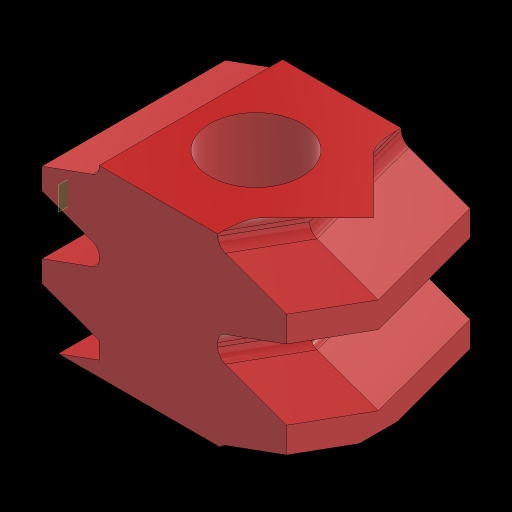
# Autodesk Inventor part: rack
Saved by Autodesk Inventor 2023.2 (Build 272271030, 271C)
## iProperties
Created: 2023-10-23
Part Number: rack
Material: Generic
Document SubType Name: Modeling
Designer: robpl
Density: 1 g/cm^3
Appearance: Red
Author: robpl
## iProperties of the stored document rack_3DPrint.ipt
Created: 2023-10-23
Part Number: rack_3DPrint
Material: Generic
Document SubType Name: Modeling
Designer: robpl
Density: 1 g/cm^3
Appearance: Default
Author: robpl
Autodesk Inventor part; units mm, degrees
ref_plane "YZ Plane" through (0, 0, 0) normal (1, 0, 0) x (0, 1, 0)
ref_plane "XZ Plane" through (0, 0, 0) normal (0, 1, 0) x (-1, 0, 0)
ref_plane "XY Plane" through (0, 0, 0) normal (0, 0, 1) x (1, 0, 0)
sketch "Sketch1" plane through (0, 0, 0) normal (0, 0, 1) x (1, 0, 0)
  line L0 (-6, -4.5) -> (6, -4.5)
  line L1 (6, -4.5) -> (6, 4.5)
  line L2 (6, 4.5) -> (-6, 4.5)
  line L3 (-6, 4.5) -> (-6, -4.5)
  point P0 (0, 0)
  point P1 (-6, 0)
  point P2 (0, 4.5)
  dimension "d0" = 12
  dimension "d1" = 9
  constraints: 8 end point, 2 midpoint, 2 parallel, 1 horizontal, 1 horizontal alignment, 1 perpendicular, 1 vertical alignment
  measures "d0" distance of L2.end L1.end
  measures "d1" distance of L1.end L0.end
extrude "Extrusion1" add sketch "Sketch1" along normal blind 4.5
sketch "Sketch2" plane through (0, 0, 4.5) normal (0, 0, 1) x (1, 0, 0)
  line L0 (6, -4.5) -> (6, 4.5) projected
  line L1 (6, 4.5) -> (-6, 4.5) projected
  line L2 (-6, 4.5) -> (-6, -4.5) projected
  line L3 (-6, -4.5) -> (6, -4.5) projected
  line L4 (6, -4.5) -> (6, 4.5) projected
  line L5 (6, 6.2241) -> (2.625, 4.9957)
  line L6 (2.625, 4.9957) -> (2.625, 4.0043)
  line L7 (2.625, 4.0043) -> (6, 2.7759)
  line L8 (6, 1.5117) -> (2.625, 0.2833)
  line L9 (2.625, 0.2833) -> (2.625, -0.708)
  line L10 (2.625, -0.708) -> (6, -1.9364)
  arc A0 (3, 5.1322) -> (2.625, 4.5965) centre (3.195, 4.5965) ccw
  arc A1 (2.625, 4.4035) -> (3, 3.8678) centre (3.195, 4.4035) ccw
  line L11 (6, 4.5) -> (-6, 4.5) projected
  arc A2 (2.625, -0.3089) -> (3, -0.8445) centre (3.195, -0.3089) ccw
  arc A3 (3, 0.4198) -> (2.625, -0.1159) centre (3.195, -0.1159) ccw
  line L12 (6, 6.2241) -> (6, 2.7759)
  line L13 (0, 4.5) -> (1.3125, -4.5)
  line L14 (0, -4.5) -> (6, -4.5) projected
  line L15 (-6.2425, 4.4387) -> (-2.6572, 4.2253)
  line L16 (-2.6572, 4.2253) -> (-2.3741, 3.2753)
  line L17 (-2.3741, 3.2753) -> (-5.2577, 1.1342)
  arc A4 (-2.5432, 3.8428) -> (-3.0556, 4.249) centre (-3.0895, 3.68) ccw
  arc A5 (-2.6946, 3.0374) -> (-2.4881, 3.6578) centre (-3.0344, 3.495) ccw
  line L18 (-6.2425, 4.4387) -> (-5.2577, 1.1342)
  line L19 (-4.8967, -0.0774) -> (-1.3114, -0.2908)
  line L20 (-1.3114, -0.2908) -> (-1.0283, -1.2408)
  line L21 (-1.0283, -1.2408) -> (-3.9119, -3.3819)
  arc A6 (-1.3487, -1.4787) -> (-1.1423, -0.8583) centre (-1.6885, -1.0211) ccw
  arc A7 (-1.1974, -0.6733) -> (-1.7098, -0.2671) centre (-1.7437, -0.8361) ccw
  point P0 (0, 0)
  point P1 (0, 0)
  point P2 (2.625, 4.5)
  point P3 (4.5, 3.3219)
  point P4 (4.5, 0.9657)
  point P5 (6, 2.7759)
  point P6 (2.625, 4.5)
  point P7 (6, -1.9364)
  point P8 (6, 1.5117)
  point P9 (6, 4.5)
  point P10 (-2.5157, 3.7503)
  point P11 (-3.9761, 2.0858)
  point P12 (-6, 3.625)
  point P13 (0, 7.2759)
  point P14 (-3.3032, -0.1723)
  point P15 (0, 2.5636)
  point P16 (0, 6.0117)
  point P17 (4.5, -1.3905)
  dimension "d14" = 70
  dimension "d15" = 4.7124
  dimension "d16" = 0.57
  dimension "d17" = 3.375
  dimension "d18" = 1.5
  dimension "d19" = 2.3562
  dimension "d48" = 2.3562
  constraints: 30 end point, 26 point on line, 23 symmetric about line, 16 point on circle, 8 centre point, 8 tangent, 4 equal length, 3 equal radius, 2 midpoint, 2 vertical, 2 vertical alignment, 1 parallel, 6 other
  measures "d14" angle of L0 L5
  measures "d15" distance of L10.end L7.end
  measures "d16" radius of A0
  measures "d17" distance between parallel lines of L6 L0
  measures "d18" distance from line of L0 point (4.5, 3.322)
  measures "d19" distance of point (4.5, 3.322) point (4.5, 0.966)
  measures "d48" distance of point (4.5, 0.966) point (4.5, -1.39)
sketch "Sketch3" plane through (6, -4.5, 0) normal (1, 0, 0) x (0, 0, -1)
  line L0 (-4.5, 0) -> (-4.5, 9) projected
  line L1 (-4.5, 9) -> (-4.5, 0) projected
  line L2 (-4.5, 2.5636) -> (0, 0.9257)
  line L3 (0, 4.5) -> (0, 9) projected
  line L4 (0, 9) -> (-4.5, 9) projected
  dimension "d31" = 20
  constraints: 2 end point, 1 point on line
  measures "d31" angle of L4 L2
sweep "Sweep1" cut profiles "Sketch2" path "Sketch3" path curves L2 contours L10 A2 L9 A3 L8 L0 | L7 A1 L6 L1 L0 | L6 A0 L5 L12 L1
pattern_linear "Rectangular Pattern2" count 8 spacing 4.7124 along (0, -1, 0) of "Sweep1"
mirror "Mirror2" about plane through (0, 0, 0) normal (0, 0, -1)
ref_plane "Work Plane3" through (4.5, 2.8745, 4.5) normal (1, 0, 0) x (0, 0, -1)
sketch "Sketch6" plane through (0, 0, 4.5) normal (0, 0, 1) x (1, 0, 0)
  arc A0 (3, -4.2926) -> (2.729, -4.5) centre (3.195, -4.8283) ccw projected
  line L0 (3, -4.2926) -> (6, -3.2007) projected
  line L1 (6, -3.2007) -> (6, -1.9364) projected
  line L2 (6, -1.9364) -> (3, -0.8445) projected
  arc A1 (2.625, -0.3089) -> (3, -0.8445) centre (3.195, -0.3089) ccw projected
  line L3 (2.625, -0.3089) -> (2.625, -0.1159) projected
  arc A2 (3, 0.4198) -> (2.625, -0.1159) centre (3.195, -0.1159) ccw projected
  line L4 (3, 0.4198) -> (6, 1.5117) projected
  line L5 (6, 1.5117) -> (6, 2.7759) projected
  line L6 (6, 2.7759) -> (3, 3.8678) projected
  arc A3 (2.625, 4.4035) -> (3, 3.8678) centre (3.195, 4.4035) ccw projected
  line L7 (2.625, 4.4035) -> (2.625, 4.5) projected
  line L8 (2.625, 4.5) -> (-6, 4.5) projected
  line L9 (-6, 4.5) -> (-6, -4.5) projected
  line L10 (-6, -4.5) -> (2.729, -4.5) projected
  line L11 (-6, 3.0633) -> (-3.1875, 4.087)
  line L12 (-3.1875, 4.087) -> (-3.1875, 4.913)
  line L13 (2.625, 4.5) -> (-6, 4.5) projected
  line L14 (-3.1875, 4.913) -> (-6, 5.9367)
  line L15 (-6, 5.9367) -> (-6, 4.5)
  arc A4 (-3.5, 3.9732) -> (-3.1875, 4.4196) centre (-3.6625, 4.4196) ccw
  arc A5 (-3.1875, 4.5804) -> (-3.5, 5.0268) centre (-3.6625, 4.5804) ccw
  arc A6 (-3.5, 0.0462) -> (-3.1875, 0.4926) centre (-3.6625, 0.4926) ccw
  line L16 (-3.1875, 0.16) -> (-3.1875, 0.9861)
  arc A7 (-3.1875, 0.6535) -> (-3.5, 1.0998) centre (-3.6625, 0.6535) ccw
  line L17 (-3.1875, 0.9861) -> (-6, 2.0097)
  line L18 (-6, 2.0097) -> (-6, 0.573)
  line L19 (-6, -0.8637) -> (-3.1875, 0.16)
  arc A8 (-3.5, -3.8808) -> (-3.1875, -3.4344) centre (-3.6625, -3.4344) ccw
  line L20 (-3.1875, -3.767) -> (-3.1875, -2.9409)
  arc A9 (-3.1875, -3.2735) -> (-3.5, -2.8272) centre (-3.6625, -3.2735) ccw
  line L21 (-3.1875, -2.9409) -> (-6, -1.9173)
  line L22 (-6, -1.9173) -> (-6, -3.354)
  line L23 (-6, -4.7907) -> (-3.1875, -3.767)
  arc A10 (-3.5, -7.8078) -> (-3.1875, -7.3614) centre (-3.6625, -7.3614) ccw
  line L24 (-3.1875, -7.694) -> (-3.1875, -6.8679)
  arc A11 (-3.1875, -7.2005) -> (-3.5, -6.7542) centre (-3.6625, -7.2005) ccw
  line L25 (-3.1875, -6.8679) -> (-6, -5.8443)
  line L26 (-6, -5.8443) -> (-6, -7.281)
  line L27 (-6, -8.7177) -> (-3.1875, -7.694)
  point P0 (0, 0)
  point P1 (-4.75, 5.4817)
  point P2 (-4.75, 3.5183)
  point P3 (-3.1875, 4.5)
  point P4 (-3.1875, 0.573)
  point P5 (-4.75, 1.5548)
  point P6 (-4.75, -0.4087)
  point P7 (-3.1875, -3.354)
  point P8 (-4.75, -2.3722)
  point P9 (-4.75, -4.3357)
  point P10 (-3.1875, -7.281)
  point P11 (-4.75, -6.2992)
  point P12 (-4.75, -8.2627)
  point P13 (-6, -0.8637)
  point P14 (-6, 2.0097)
  point P15 (-5.2013, -4.5)
  point P16 (-6, -1.9173)
  dimension "d50" = 70
  dimension "d51" = 1.25
  dimension "d52" = 1.5625
  dimension "d53" = 1.9635
  dimension "d54" = 0.475
  dimension "d57" = 3.927
  constraints: 32 end point, 26 point on line, 16 point on circle, 8 centre point, 4 tangent, 1 equal length, 1 equal radius, 1 midpoint, 1 parallel, 1 perpendicular, 1 vertical, 1 vertical alignment, 60 other
  measures "d50" angle of L15 L14
  measures "d51" distance from line of L15 point (-4.75, 5.482)
  measures "d52" distance from line of point (-4.75, 5.482) L12
  measures "d53" distance of point (-4.75, 3.518) point (-4.75, 5.482)
  measures "d54" radius of A5
  measures "d57" distance of L11.end L16.start
extrude "Extrusion4" cut sketch "Sketch6" against normal blind 10 contours L10 L9 L21 A9 L20 A8 L23 | A8 L20 L23 | A9 L21 L20 | L9 L17 A7 L16 A6 L19 | L9 L8 L12 A4 L11
ref_plane "Work Plane4" through (-4.75, 2.0097, -4.5) normal (-1, 0, 0) x (0, 0, 1)
sketch "Sketch7" plane through (0, 0, 0) normal (0, 1, 0) x (-1, 0, 0)
  circle A0 centre (0, 0) radius 2.25
  dimension "d65" = 4.5
  constraints: 2 coincident, 1 centre point
  measures "d65" diameter of A0
extrude "Extrusion5" cut sketch "Sketch7" along normal through all both and the other way through all
equation "\"d15\" = 3.14159 * d18"
equation "\"d16\" = 0.38 * d18"
equation "\"d17\" = 2.25 * d18"
equation "\"d19\" = 0.5 * d15"
equation "\"d48\" = d19"
equation "\"d52\" = 1.25 * d51"
equation "\"d53\" = 1.5708 * d51"
equation "\"d54\" = 0.38 * d51"
equation "\"d57\" = 3.14159 * d51"
equation "\"d32\" = 20.5deg"
body "Solid1"
